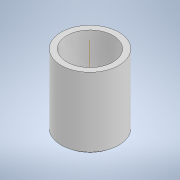
# Autodesk Inventor part: 2020-simulatedFilterWithThread
Saved by Autodesk Inventor 2020.2 (Build 242310000, 310)
## iProperties
Created: 2020-04-14
Part Number: 2020-simulatedFilterWithThread
Material: Generic
Document SubType Name: Modeling
Designer: robst
Density: 1 g/cm^3
Appearance: Default
Author: robst
Autodesk Inventor part; units mm, degrees
ref_plane "YZ Plane" through (0, 0, 0) normal (1, 0, 0) x (0, 1, 0)
ref_plane "XZ Plane" through (0, 0, 0) normal (0, 1, 0) x (-1, 0, 0)
ref_plane "XY Plane" through (0, 0, 0) normal (0, 0, 1) x (1, 0, 0)
sketch "Sketch1" plane through (0, 0, 0) normal (0, 0, 1) x (1, 0, 0)
  line L0 (28.575, 0) -> (28.575, 2.54)
  line L1 (28.575, 2.54) -> (31.75, 2.54)
  line L2 (31.75, 2.54) -> (31.75, 78.74)
  line L3 (31.75, 78.74) -> (25.4, 78.74)
  line L4 (25.4, 78.74) -> (25.4, 0)
  line L5 (25.4, 0) -> (28.575, 0)
  line L6 (0, -15.748) -> (0, 94.488) projected
  point P0 (0, 0)
  dimension "d0" = 31.75
  dimension "d1" = 28.575
  dimension "d2" = 25.4
  dimension "d3" = 2.54
  dimension "d4" = 76.2
  constraints: 12 end point, 4 perpendicular, 1 horizontal, 1 vertical
  measures "d0" distance from line of point (0, 0) L2
  measures "d1" distance from line of point (0, 0) L0
  measures "d2" distance from line of point (0, 0) L4
  measures "d3" distance of L0.end L0.start
  measures "d4" distance of L2.end L1.end
revolve "Revolution1" add sketch "Sketch1" angle 360 about axis through (0, -10, 0) along (0, 1, 0)
body "Solid1"
